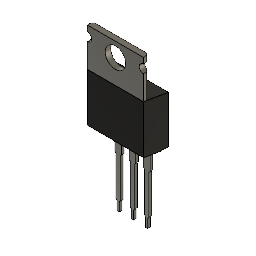
335 MOSFET N-channel (Autodesk Fusion 360 design; units mm, degrees)
Autodesk Fusion 360 part; units mm, degrees
sketch "Sketch2" plane through (0, 0, 0) normal (0, 1, 0) x (1, 0, 0)
  line L0 (5, -8) -> (-5, -8)
  line L1 (-5, -8) -> (-5, 8)
  line L2 (-5, 8) -> (5, 8)
  line L3 (5, 8) -> (5, -8)
  line L4 (5, -8) -> (-5, 8) construction
  line L5 (-5, -8) -> (5, 8) construction
  circle A0 centre (0, -5.46) radius 1.8
  line L6 (-5, 8) -> (5, 8)
  line L7 (5, 8) -> (5, -1)
  line L8 (5, -1) -> (-5, -1)
  line L9 (-5, -1) -> (-5, 8)
  circle A1 centre (-5, -6.22) radius 0.76
  circle A2 centre (5, -6.22) radius 0.76
  line L10 (-2.5112, 8) -> (-2.5112, 21) construction
  line L11 (-3.1112, 8) -> (-3.1112, 12)
  line L12 (-3.1112, 12) -> (-2.9112, 12.2)
  line L13 (-2.9112, 12.2) -> (-2.9112, 19.2)
  line L14 (-2.9112, 19.2) -> (-2.7112, 19.4)
  line L15 (-2.7112, 19.4) -> (-2.7112, 21)
  line L16 (-2.7112, 21) -> (-2.5112, 21)
  line L17 (-1.9112, 8) -> (-1.9112, 12)
  line L18 (-1.9112, 12) -> (-2.1112, 12.2)
  line L19 (-2.1112, 12.2) -> (-2.1112, 19.2)
  line L20 (-2.1112, 19.2) -> (-2.3112, 19.4)
  line L21 (-2.3112, 19.4) -> (-2.3112, 21)
  line L22 (-2.3112, 21) -> (-2.5112, 21)
  dimension "d1" = 10
  dimension "d2" = 16
  dimension "d3" = 3.6
  dimension "d4" = 2.54
  dimension "d5" = 10
  dimension "d6" = 9
  dimension "d7" = 1.52
  dimension "d8" = 1.78
  dimension "d9" = 1.52
  dimension "d10" = 1.78
  dimension "d11" = 13
  dimension "d12" = 135
  dimension "d13" = 0.6
  dimension "d14" = 0.4
  dimension "d15" = 135
  dimension "d16" = 0.2
  dimension "d17" = 4
  dimension "d18" = 7
  measures "d3" diameter of A0
  measures "d4" distance of L0
  measures "d7" diameter of A1
  measures "d9" diameter of A2
  measures "d12" angle of L11 L12
  measures "d13" distance of L10 L11
  measures "d14" distance of L10 L13
  measures "d15" angle of L13 L14
  measures "d16" distance of L10 L15
extrude "Extrude1" add sketch "Sketch2" along normal blind 0.5 from surface at 3 contours L2 L6 L11 L12 L13 L14 L15 L16 L17 L18 L19 L20 L21 L22 makes body 1
pattern_linear "R-Pattern1" count 3 spacing 2.54 along (1, 0, 0) of bodies 1 makes body 2 at (0.2288, 3, -9.3333) makes body 3 at (2.7688, 3, -9.3333)
extrude "Extrude2" add sketch "Sketch2" along normal blind 1 separate body contours L0 L1 L3 L8 A1 A2 makes body 4
extrude "Extrude3" add sketch "Sketch2" along normal blind 4.5 separate body contours L1 L2 L3 L6 L7 L8 L9 makes body 5
draft "Draft1" angle 10 neutral plane through (0, 1, 0) pull (0, 1, 0) 1 faces at (1.6667, 1.5, 1) on bodies 5
draft "Draft2" angle -10 neutral plane through (0, 1, 0) pull (0, 1, 0) 1 faces at (1.6667, 0.3333, 1) on bodies 4
chamfer "Chamfer1" distance 0.4 angle 45 4 edges at (5, 1, 7.49) (5, 1, 3.23) (-5, 1, 7.49) (-5, 1, 3.23) on bodies 4
sketch "Sketch3" plane through (0, 0, 0) normal (1, 0, 0) x (0, 1, 0)
  line L0 (0, -8) -> (4.5, -8)
  line L1 (0, 1.1763) -> (0, -8)
  line L2 (3, -8) -> (0, -7.471)
  dimension "d36" = 10
  dimension "d37" = 1.5
  measures "d36" angle of L0 L2
extrude "Extrude4" cut sketch "Sketch3" along normal mid plane 18.6 bodies 5
equation "d7 = ( 0.76 * 2 ) * 1 mm"
equation "d8 = 2.54 mm - 0.76 mm"
